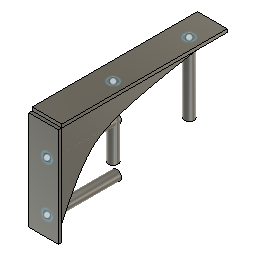
Main v9 (Autodesk Fusion 360 design; units mm, degrees)
Autodesk Fusion 360 part; units mm, degrees
sketch "Sketch1" plane through (0, 0, 0) normal (1, 0, 0) x (0, 1, 0)
  line L0 (0, 0) -> (0, 150)
  line L1 (0, 150) -> (250, 150)
  line L2 (0, 150) -> (125, 25) construction
  line L3 (250, 150) -> (250, 140)
  line L4 (0, 0) -> (10, 0)
  spline S0 degree 5 poles (10, 0) (12.7675, 5.9452) (18.1969, 17.4133) (26.0252, 33.3492) (35.807, 52.0174) (47.3001, 70.9752) (59.009, 85.6945) (73.4467, 97.0686) (93.9845, 106.6977) (121.6234, 115.3853) (156.7317, 123.6963) (190.5953, 130.2378) (219.1077, 135.1262) (239.4759, 138.3768) (250, 140) knots 0 0 0 0 0 0 0.1 0.2 0.3 0.4 0.5 0.6 0.7 0.8 0.9 1 1 1 1 1 1
  line L5 (47.5613, 74.1192) -> (77.4387, 100.8808)
  point P0 (62.5, 87.5)
  dimension "d1" = 150
  dimension "d2" = 250
  constraint coincident L0.start L4.start
  constraint vertical L0
  constraint perpendicular L0 L1
  constraint perpendicular L1 L3
  constraint perpendicular L0 L4
  constraint midpoint L2 P0
  constraint midpoint P0 L5
  measures "d1" distance of L0.start L0.end
  measures "d2" distance of L0.end L1.end
extrude "Extrude1" add sketch "Sketch1" along normal blind 15 makes body 1
sketch "Sketch2" plane through (0, 0, 150) normal (0, 0, 1) x (-1, 0, 0)
  line L0 (0, -250) -> (0, 0)
  line L1 (0, 0) -> (-15, 0)
  line L2 (-15, 0) -> (-15, -250)
  line L3 (-15, -250) -> (0, -250)
  line L4 (0, 0) -> (-15, 0)
  line L5 (-15, 0) -> (-15, -250)
  line L6 (0, -250) -> (0, 0)
  line L7 (0, -250) -> (-15, -250)
  constraint coincident L0.end L1.start
  constraint coincident L1.end L2.start
  constraint coincident L2.end L3.start
  constraint coincident L0.start L3.end
sketch "Sketch3" plane through (0, 0, 0) normal (0, -1, 0) x (1, 0, 0)
  line L0 (0, 150) -> (0, 0)
  line L1 (0, 0) -> (15, 0)
  line L2 (15, 0) -> (15, 150)
  line L3 (15, 150) -> (0, 150)
  line L4 (0, 150) -> (15, 150)
  line L5 (15, 0) -> (0, 0)
  line L6 (15, 150) -> (15, 0)
  constraint coincident L0.start L3.end
  constraint coincident L2.end L3.start
  constraint coincident L1.end L2.start
  constraint coincident L0.end L1.start
sketch "Sketch4" plane through (0, 0, 150) normal (0, 0, 1) x (-1, 0, 0)
  circle A0 centre (-7.5, -215) radius 7.5
  circle A1 centre (-7.5, -215) radius 2.5
  constraint concentric A0 A1
sketch "Sketch8" plane through (0, 0, 150) normal (0, 0, 1) x (1, 0, 0)
  circle A0 centre (7.5, 100) radius 7.5
  circle A1 centre (7.5, 100) radius 2.5
  constraint concentric A0 A1
extrude "Extrude2" add sketch "Sketch4" against normal blind 5 separate body makes body 2
extrude "Extrude3" add sketch "Sketch8" against normal blind 5 separate body makes body 3
sketch "Sketch9" plane through (0, 0, 0) normal (0, -1, 0) x (1, 0, 0)
  circle A0 centre (7.5, 25) radius 7.5
  circle A1 centre (7.5, 25) radius 2.5
  circle A2 centre (7.5, 100) radius 7.5
  circle A3 centre (7.5, 100) radius 2.5
  dimension "d10" = 15
  constraint concentric A0 A1
  constraint concentric A2 A3
  measures "d10" diameter of A0
extrude "Extrude4" add sketch "Sketch9" against normal blind 5 separate body contours A0 makes body 4
extrude "Extrude5" add sketch "Sketch9" against normal blind 5 separate body contours A2 makes body 5
extrude "Extrude1'" add sketch "Sketch3" along normal blind 5 separate body makes body 6 in component "Vägg"
extrude "Extrude2'" add 1 faces at (0, -1.6667, 100) along direction (-1, 0, 0) blind 15 on bodies 6 bodies 6 in component "Vägg"
extrude "Extrude3'" add 1 faces at (15, -1.6667, 50) along direction (1, 0, 0) blind 15 on bodies 6 bodies 6 in component "Vägg"
extrude "Extrude1''" add sketch "Sketch2" along normal blind 5 separate body makes body 7 in component "Hyllplan"
extrude "Extrude2''" add 1 faces at (15, 83.3333, 151.6667) along direction (1, 0, 0) blind 15 on bodies 7 bodies 7 in component "Hyllplan"
extrude "Extrude3''" add 1 faces at (0, 166.6667, 151.6667) along direction (-1, 0, 0) blind 15 on bodies 7 bodies 7 in component "Hyllplan"
sketch "Sketch10" plane through (0, 5, 0) normal (0, 1, 0) x (-1, 0, 0)
  circle A0 centre (-7.5, 25) radius 2.5
  circle A1 centre (-7.5, 25) radius 7.5
  circle A2 centre (-7.5, 25) radius 7.5
  constraint tangent A1 A2
extrude "Extrude1'''" add sketch "Sketch10" along normal blind 100 separate body makes body 8 in component "SkruvClearance"
extrude "Extrude2'''" add sketch "Sketch9" against normal blind 105 contours A1 bodies 8 in component "SkruvClearance"
extrude "Extrude1''''" add 1 faces at (13.2961, 5, 99.5032) along direction (0, 1, 0) blind 100 separate body on bodies 5 makes body 9 in component "SkruvClearance (1)"
extrude "Extrude2''''" add sketch "Sketch9" against normal blind 105 contours A3 bodies 9 in component "SkruvClearance (1)"
extrude "Extrude1'''''" add 1 faces at (13.2961, 99.5032, 145) along direction (0, 0, -1) blind 100 separate body on bodies 3 makes body 10 in component "SkruvClearance (2)"
extrude "Extrude2'''''" add sketch "Sketch8" against normal blind 105 contours A1 bodies 10 in component "SkruvClearance (2)"
extrude "Extrude1''''''" add 1 faces at (1.8427, 213.6449, 145) along direction (0, 0, -1) blind 100 separate body on bodies 2 makes body 11 in component "SkruvClearance (3)"
extrude "Extrude2''''''" add sketch "Sketch4" against normal blind 105 contours A1 bodies 11 in component "SkruvClearance (3)"
component "Vägg" placed x (1, 0, 0) y (0, 1, 0) z (0, 0, 1) at (0, 0, 0)
component "Hyllplan" placed x (1, 0, 0) y (0, 1, 0) z (0, 0, 1) at (0, 0, 0)
component "SkruvClearance" placed x (1, 0, 0) y (0, 1, 0) z (0, 0, 1) at (0, 0, 0)
component "SkruvClearance (1)" placed x (1, 0, 0) y (0, 1, 0) z (0, 0, 1) at (0, 0, 0)
component "SkruvClearance (2)" placed x (1, 0, 0) y (0, 1, 0) z (0, 0, 1) at (0, 0, 0)
component "SkruvClearance (3)" placed x (1, 0, 0) y (0, 1, 0) z (0, 0, 1) at (0, 0, 0)
